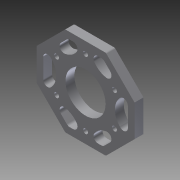
# Autodesk Inventor part: lower box upper plate 2
Saved by Autodesk Inventor 2012 (Build 160160000, 160)
## iProperties
Created: 2013-08-26
Part Number: lower box upper plate 2
Material: Default
Document SubType Name: Modeling
Designer: Bryce
Density: 1 g/cm^3
Author: Bryce
Autodesk Inventor part; units mm, degrees
ref_plane "YZ Plane" through (0, 0, 0) normal (1, 0, 0) x (0, 1, 0)
ref_plane "XZ Plane" through (0, 0, 0) normal (0, 1, 0) x (-1, 0, 0)
ref_plane "XY Plane" through (0, 0, 0) normal (0, 0, 1) x (1, 0, 0)
sketch "Sketch1" plane through (0, 0, 0) normal (0, 0, 1) x (1, 0, 0)
  line L0 (-34.925, 31.75) -> (-14.4664, 31.75) construction
  line L1 (34.925, 31.75) -> (34.925, 11.2914) construction
  line L2 (34.925, -31.75) -> (14.4664, -31.75) construction
  line L3 (-34.925, -31.75) -> (-34.925, -11.2914) construction
  line L4 (-34.925, -11.2914) -> (-14.4664, -31.75)
  line L5 (14.4664, -31.75) -> (34.925, -11.2914)
  line L6 (34.925, 11.2914) -> (14.4664, 31.75)
  line L7 (-14.4664, 31.75) -> (-34.925, 11.2914)
  line L8 (-34.925, 11.2914) -> (-34.925, 31.75) construction
  line L9 (-14.4664, 31.75) -> (14.4664, 31.75)
  line L10 (14.4664, 31.75) -> (34.925, 31.75) construction
  line L11 (34.925, 11.2914) -> (34.925, -11.2914)
  line L12 (34.925, -11.2914) -> (34.925, -31.75) construction
  line L13 (14.4664, -31.75) -> (-14.4664, -31.75)
  line L14 (-14.4664, -31.75) -> (-34.925, -31.75) construction
  line L15 (-34.925, -11.2914) -> (-34.925, 11.2914)
  circle A0 centre (0, 23.8252) radius 1.7272
  circle A1 centre (0, 0) radius 14.2875
  circle A2 centre (-20.6332, 11.9126) radius 1.7272
  circle A3 centre (-20.6332, -11.9126) radius 1.7272
  circle A4 centre (0, -23.8252) radius 1.7272
  circle A5 centre (20.6332, -11.9126) radius 1.7272
  circle A6 centre (20.6332, 11.9126) radius 1.7272
  line L16 (-12.4937, -26.9875) -> (12.4937, -26.9875)
  line L17 (12.4937, -26.9875) -> (17.5499, -21.9313)
  line L18 (30.1625, -9.3187) -> (30.1625, 9.3187)
  line L19 (30.1625, 9.3187) -> (29.6813, 9.7999)
  line L20 (12.4937, 26.9875) -> (-12.4937, 26.9875)
  line L21 (-12.4937, 26.9875) -> (-17.5499, 21.9313)
  line L22 (-30.1625, 9.3187) -> (-30.1625, -9.3187)
  line L23 (-30.1625, -9.3187) -> (-29.6813, -9.7999)
  arc A7 (-24.1009, -15.3803) -> (-19.5646, -16.6988) centre (-20.6332, -11.9126) ccw construction
  arc A8 (-4.6793, -25.2929) -> (-14.8073, -16.5505) centre (-16.7972, -29.0936) ccw
  arc A9 (-24.2439, -8.594) -> (-24.7627, -9.2674) centre (-20.6332, -11.9126) ccw
  arc A10 (-24.1009, 15.3803) -> (-24.7627, 9.2674) centre (-20.6332, 11.9126) ccw construction
  arc A11 (-24.2439, -8.594) -> (-24.2439, 8.594) centre (-33.5944, 0) ccw
  arc A12 (-19.5646, 16.6988) -> (-24.1009, 15.3803) centre (-20.6332, 11.9126) ccw construction
  arc A13 (-3.7483, 26.9875) -> (-4.6793, 25.2929) centre (0, 23.8252) ccw
  arc A14 (4.6793, 25.2929) -> (3.7483, 26.9875) centre (0, 23.8252) ccw
  arc A15 (-4.6793, -25.2929) -> (-3.7483, -26.9875) centre (0, -23.8252) ccw
  arc A16 (3.7483, -26.9875) -> (4.6793, -25.2929) centre (0, -23.8252) ccw
  arc A17 (24.1009, 15.3803) -> (19.5646, 16.6988) centre (20.6332, 11.9126) ccw construction
  arc A18 (24.2439, 8.594) -> (24.7627, 9.2674) centre (20.6332, 11.9126) ccw
  arc A19 (24.1009, -15.3803) -> (24.7627, -9.2674) centre (20.6332, -11.9126) ccw construction
  arc A20 (19.5646, -16.6988) -> (24.1009, -15.3803) centre (20.6332, -11.9126) ccw construction
  arc A21 (-19.5646, 16.6988) -> (-14.8073, 16.5505) centre (-16.7972, 29.0936) ccw construction
  arc A22 (4.6793, 25.2929) -> (14.8073, 16.5505) centre (16.7972, 29.0936) ccw
  arc A23 (19.5646, -16.6988) -> (14.8073, -16.5505) centre (16.7972, -29.0936) ccw construction
  arc A24 (24.2439, 8.594) -> (24.2439, -8.594) centre (33.5944, 0) ccw
  arc A25 (-24.7627, 9.2674) -> (-29.6813, 9.7999) centre (-27.4363, 7.5548) ccw
  arc A26 (-17.5499, 21.9313) -> (-14.8073, 16.5505) centre (-15.3048, 19.6863) ccw
  arc A27 (-24.7627, 9.2674) -> (-24.2439, 8.594) centre (-20.6332, 11.9126) ccw
  line L24 (-29.6813, 9.7999) -> (-30.1625, 9.3187)
  line L25 (-17.5499, 21.9313) -> (-29.6813, 9.7999) construction
  arc A28 (-14.8073, 16.5505) -> (-4.6793, 25.2929) centre (-16.7972, 29.0936) ccw
  arc A29 (-29.6813, -9.7999) -> (-24.7627, -9.2674) centre (-27.4363, -7.5548) ccw
  arc A30 (-14.8073, -16.5505) -> (-17.5499, -21.9313) centre (-15.3048, -19.6863) ccw
  arc A31 (17.5499, -21.9313) -> (14.8073, -16.5505) centre (15.3048, -19.6863) ccw
  arc A32 (24.7627, -9.2674) -> (29.6813, -9.7999) centre (27.4363, -7.5548) ccw
  arc A33 (29.6813, 9.7999) -> (24.7627, 9.2674) centre (27.4363, 7.5548) ccw
  arc A34 (14.8073, 16.5505) -> (17.5499, 21.9313) centre (15.3048, 19.6863) ccw
  line L26 (-29.6813, -9.7999) -> (-17.5499, -21.9313) construction
  line L27 (-17.5499, -21.9313) -> (-12.4937, -26.9875)
  arc A35 (-14.8073, -16.5505) -> (-19.5646, -16.6988) centre (-16.7972, -29.0936) ccw construction
  arc A36 (-24.7627, -9.2674) -> (-24.1009, -15.3803) centre (-20.6332, -11.9126) ccw construction
  arc A37 (14.8073, -16.5505) -> (4.6793, -25.2929) centre (16.7972, -29.0936) ccw
  line L28 (17.5499, -21.9313) -> (29.6813, -9.7999) construction
  line L29 (29.6813, -9.7999) -> (30.1625, -9.3187)
  arc A38 (24.7627, -9.2674) -> (24.2439, -8.594) centre (20.6332, -11.9126) ccw
  arc A39 (24.7627, 9.2674) -> (24.1009, 15.3803) centre (20.6332, 11.9126) ccw construction
  line L30 (29.6813, 9.7999) -> (17.5499, 21.9313) construction
  arc A40 (14.8073, 16.5505) -> (19.5646, 16.6988) centre (16.7972, 29.0936) ccw construction
  line L31 (17.5499, 21.9313) -> (12.4937, 26.9875)
  dimension "d0" = 69.85
  dimension "d1" = 63.5
  dimension "d2" = 34.925
  dimension "d3" = 31.75
  dimension "d6" = 45
  dimension "d7" = 45
  dimension "d8" = 45
  dimension "d10" = 3.4544
  dimension "d11" = 23.8252
  dimension "d18" = 28.575
  dimension "d22" = 360
  dimension "d24" = 4.7625
  dimension "d25" = 4.7625
  dimension "d26" = 4.7625
  dimension "d27" = 4.7625
  dimension "d28" = 4.7625
  dimension "d29" = 4.7625
  dimension "d30" = 4.7625
  dimension "d32" = 4.7625
  dimension "d33" = 12.7
  dimension "d39" = 3.175
  constraints: 68 point on circle, 64 end point, 47 tangent, 41 centre point, 32 parallel, 19 equal radius, 18 point on line, 12 coincident, 11 perpendicular, 5 equal length, 3 horizontal, 1 vertical alignment, 13 other
  measures "d0" distance of L0.start L1.start
  measures "d1" distance of L1.start L2.start
  measures "d2" distance from line of L3 point (0, 0)
  measures "d3" distance from line of L2 point (0, 0)
  measures "d6" angle of L14 L4
  measures "d7" angle of L2 L5
  measures "d8" angle of L0 L7
  measures "d10" diameter of A0
  measures "d11" distance of point (0, 0) A0.centre
  measures "d18" diameter of A1
  measures "d24" distance between parallel lines of L15 L22
  measures "d25" distance between parallel lines of L4 L23
  measures "d26" distance between parallel lines of L13 L16
  measures "d27" distance between parallel lines of L5 L17
  measures "d28" distance between parallel lines of L11 L18
  measures "d29" distance between parallel lines of L6 L19
  measures "d30" distance between parallel lines of L9 L20
  measures "d32" distance between parallel lines of L7 L21
  measures "d33" radius of A21
  measures "d39" radius of A25
extrude "Extrusion1" add sketch "Sketch1" along normal blind 6.35
fillet "Fillet1" radius 3.175 12 edges at (-30.1625, 9.3187, 3.175) (-30.1625, -9.3187, 3.175) (-12.4937, 26.9875, 3.175) (-12.4937, -26.9875, 3.175) (-3.7483, 26.9875, 3.175) (-3.7483, -26.9875, 3.175) (3.7483, 26.9875, 3.175) (3.7483, -26.9875, 3.175) (12.4937, 26.9875, 3.175) (12.4937, -26.9875, 3.175) (30.1625, 9.3187, 3.175) (30.1625, -9.3187, 3.175)
fillet "Fillet2" radius 1.5875 4 edges at (-14.4664, -31.75, 3.175) (14.4664, -31.75, 3.175) (-14.4664, 31.75, 3.175) (14.4664, 31.75, 3.175)
equation "\"d2\" = 0.5 * d0"
equation "\"d3\" = 0.5 * d1"
equation "\"d7\" = d6"
equation "\"d8\" = d6"
equation "\"d25\" = d24"
equation "\"d26\" = d25"
equation "\"d27\" = d24"
equation "\"d28\" = d24"
equation "\"d29\" = d24"
equation "\"d30\" = d24"
equation "\"d32\" = d24"
body "Solid1"
